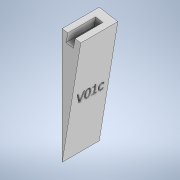
# Autodesk Inventor part: backPlateForLight
Saved by Autodesk Inventor 2021.1 (Build 251245000, 245)
## iProperties
Created: 2020-08-01
Part Number: backPlateForLight
Material: Generic
Document SubType Name: Modeling
Designer: robst
Density: 1 g/cm^3
Appearance: Default
Author: robst
Autodesk Inventor part; units mm, degrees
ref_plane "YZ Plane" through (0, 0, 0) normal (1, 0, 0) x (0, 1, 0)
ref_plane "XZ Plane" through (0, 0, 0) normal (0, 1, 0) x (-1, 0, 0)
ref_plane "XY Plane" through (0, 0, 0) normal (0, 0, 1) x (1, 0, 0)
sketch "Sketch1" plane through (0, 0, 0) normal (0, 0, 1) x (1, 0, 0)
  line L0 (0, 0) -> (0, 79.375)
  line L1 (0, 79.375) -> (12.7, 77.1356)
  line L2 (12.7, 77.1356) -> (0, 0)
  dimension "d0" = 79.375
  dimension "d6" = 80
  dimension "d8" = 12.7
  constraints: 6 end point, 1 vertical
  measures "d0" distance of L0.start L0.end
  measures "d6" angle of L1 L0
  measures "d8" distance from line of L1.end L0
extrude "Extrusion1" add sketch "Sketch1" against normal blind 25.4
sketch "Sketch4" plane through (0, 0, 0) normal (0.9867155, -0.1624578, 0) x (0, 0, -1)
  line L0 (0, 0) -> (0, 78.1742) construction
  line L1 (0, 39.0871) -> (25.4, 39.0871) construction
  line L2 (25.4, 78.1742) -> (25.4, 0) construction
  line L3 (8.5627, 42.2621) -> (6.3757, 35.9121)
  line L4 (6.3757, 35.9121) -> (5.4649, 35.9121)
  line L5 (5.4649, 35.9121) -> (3.2779, 42.2621)
  line L6 (3.2779, 42.2621) -> (4.1836, 42.2621)
  line L7 (4.1836, 42.2621) -> (5.9435, 36.9876)
  line L8 (5.9435, 36.9876) -> (7.7034, 42.2621)
  line L9 (7.7034, 42.2621) -> (8.5627, 42.2621)
  spline S0 degree 2 poles (13.0139, 39.0871) (13.0139, 37.3786) (12.0207, 35.7783) (10.9864, 35.7783) knots 0 0 0 1 2 2 2
  spline S1 degree 2 poles (10.9864, 35.7783) (9.9367, 35.7783) (8.9538, 37.4095) (8.9538, 39.0819) knots 0 0 0 1 2 2 2
  spline S2 degree 2 poles (8.9538, 39.0819) (8.9538, 40.8006) (9.947, 42.3907) (10.9864, 42.3907) knots 0 0 0 1 2 2 2
  spline S3 degree 2 poles (10.9864, 42.3907) (12.031, 42.3907) (13.0139, 40.744) (13.0139, 39.0871) knots 0 0 0 1 2 2 2
  spline S4 degree 2 poles (11.923, 37.1522) (12.0465, 37.4661) (12.1494, 38.4336) (12.1494, 39.0871) knots 0 0 0 1 2 2 2
  spline S5 degree 2 poles (12.1494, 39.0871) (12.1494, 39.7406) (12.0465, 40.7029) (11.9178, 41.0271) knots 0 0 0 1 2 2 2
  spline S6 degree 2 poles (11.9178, 41.0271) (11.7892, 41.3513) (11.3415, 41.6857) (10.9864, 41.6857) knots 0 0 0 1 2 2 2
  spline S7 degree 2 poles (10.9864, 41.6857) (10.6314, 41.6857) (10.1734, 41.3513) (10.0396, 41.0168) knots 0 0 0 1 2 2 2
  spline S8 degree 2 poles (10.0396, 41.0168) (9.9109, 40.6926) (9.8183, 39.7046) (9.8183, 39.0819) knots 0 0 0 1 2 2 2
  spline S9 degree 2 poles (9.8183, 39.0819) (9.8183, 38.413) (9.9006, 37.5176) (10.0344, 37.1677) knots 0 0 0 1 2 2 2
  spline S10 degree 2 poles (10.0344, 37.1677) (10.1579, 36.8383) (10.6159, 36.4833) (10.9864, 36.4833) knots 0 0 0 1 2 2 2
  spline S11 degree 2 poles (10.9864, 36.4833) (11.3363, 36.4833) (11.7943, 36.8177) (11.923, 37.1522) knots 0 0 0 1 2 2 2
  line L10 (17.4239, 35.9121) -> (14.3261, 35.9121)
  line L11 (14.3261, 35.9121) -> (14.3261, 36.5605)
  line L12 (14.3261, 36.5605) -> (15.4788, 36.5605)
  line L13 (15.4788, 36.5605) -> (15.4788, 40.8161)
  line L14 (15.4788, 40.8161) -> (14.3261, 40.8161)
  line L15 (14.3261, 40.8161) -> (14.3261, 41.3976)
  spline S12 degree 2 poles (14.3261, 41.3976) (14.9796, 41.3976) (15.5971, 41.7681) (15.6383, 42.2827) knots 0 0 0 1 2 2 2
  line L16 (15.6383, 42.2827) -> (16.297, 42.2827)
  line L17 (16.297, 42.2827) -> (16.297, 36.5605)
  line L18 (16.297, 36.5605) -> (17.4239, 36.5605)
  line L19 (17.4239, 36.5605) -> (17.4239, 35.9121)
  spline S13 degree 2 poles (20.6041, 35.804) (20.11, 35.804) (19.2919, 36.1076) (18.9985, 36.4164) knots 0 0 0 1 2 2 2
  spline S14 degree 2 poles (18.9985, 36.4164) (18.7052, 36.72) (18.381, 37.6565) (18.381, 38.2843) knots 0 0 0 1 2 2 2
  spline S15 degree 2 poles (18.381, 38.2843) (18.381, 38.9121) (18.7155, 39.8281) (18.9985, 40.1368) knots 0 0 0 1 2 2 2
  spline S16 degree 2 poles (18.9985, 40.1368) (19.2816, 40.4507) (20.1203, 40.7852) (20.6041, 40.7852) knots 0 0 0 1 2 2 2
  spline S17 degree 2 poles (20.6041, 40.7852) (20.9951, 40.7852) (21.7259, 40.5639) (22.0089, 40.4199) knots 0 0 0 1 2 2 2
  line L20 (22.0089, 40.4199) -> (22.0089, 39.5193)
  line L21 (22.0089, 39.5193) -> (21.9626, 39.5193)
  spline S18 degree 2 poles (21.9626, 39.5193) (21.8751, 39.5914) (21.6075, 39.7766) (21.4171, 39.8744) knots 0 0 0 1 2 2 2
  spline S19 degree 2 poles (21.4171, 39.8744) (21.2473, 39.9567) (20.7944, 40.0854) (20.5886, 40.0854) knots 0 0 0 1 2 2 2
  spline S20 degree 2 poles (20.5886, 40.0854) (19.966, 40.0854) (19.2095, 39.1437) (19.2095, 38.2843) knots 0 0 0 1 2 2 2
  spline S21 degree 2 poles (19.2095, 38.2843) (19.2095, 37.4455) (19.9402, 36.5039) (20.5886, 36.5039) knots 0 0 0 1 2 2 2
  spline S22 degree 2 poles (20.5886, 36.5039) (20.9797, 36.5039) (21.6898, 36.828) (21.9626, 37.0802) knots 0 0 0 1 2 2 2
  line L22 (21.9626, 37.0802) -> (22.0089, 37.0802)
  line L23 (22.0089, 37.0802) -> (22.0089, 36.1797)
  spline S23 degree 2 poles (22.0089, 36.1797) (21.8905, 36.1231) (21.5303, 35.9635) (21.3862, 35.9275) knots 0 0 0 1 2 2 2
  spline S24 degree 2 poles (21.3862, 35.9275) (21.1804, 35.8658) (20.8562, 35.804) (20.6041, 35.804) knots 0 0 0 1 2 2 2
  constraints: 2 end point, 2 midpoint, 1 horizontal
extrude "Extrusion4" cut sketch "Sketch4" against normal blind 2.54
sketch "Sketch5" plane through (0, 0, 0) normal (0, 0, 1) x (1, 0, 0)
  line L0 (12.7, 77.1356) -> (0, 79.375) projected
  line L1 (3.8486, 78.6964) -> (2.7459, 72.4429)
  line L2 (2.7459, 72.4429) -> (7.7487, 71.5607)
  line L3 (7.7487, 71.5607) -> (8.8514, 77.8143)
  line L4 (8.8514, 77.8143) -> (3.8486, 78.6964)
  point P0 (0, 0)
  dimension "d13" = 5.08
  dimension "d14" = 3.908
  dimension "angledHeight" = 12.8959
  dimension "d16" = 6.35
  constraints: 8 end point, 3 perpendicular, 2 point on line, 1 collinear
  measures "d13" distance of L3.end L1.start
  measures "d14" distance of L1.start L0.end
  measures "angledHeight" distance of L0.start L0.end
  measures "d16" distance of L2.end L3.end
extrude "Extrusion5" cut sketch "Sketch5" against normal blind 19.05
equation "\"d2\" = partWidth"
equation "\"d13\" = slotWidth"
equation "\"d14\" = x"
equation "\"d16\" = slotDepth"
equation "\"d17\" = slotLength"
equation "\"slotWidth\" = 5.08"
equation "\"x\" = -0.5 * slotWidth + 0.5 * angledHeight"
equation "\"slotDepth\" = 6.35"
equation "\"slotLength\" = 0.75 * partWidth"
equation "\"partWidth\" = 25.4"
body "Solid1"
